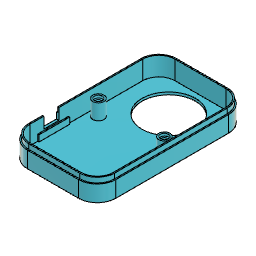
Gehaeuse_unten (Autodesk Fusion 360 design; units mm, degrees)
Autodesk Fusion 360 part; units mm, degrees
note: some values were not read from the file. Set by a fixed rule: which face or edge a step refers to.
sketch "Skizze1" plane through (0, 0, 0) normal (0, 0, 1) x (1, 0, 0)
  circle A0 centre (0, 0) radius 32.5
  circle A1 centre (0, 58.5) radius 21.5
  arc A2 (20.5, -34.5) -> (35.5, -19.5) centre (20.5, -19.5) ccw
  line L0 (35.5, -19.5) -> (35.5, 71)
  arc A3 (35.5, 71) -> (20.5, 86) centre (20.5, 71) ccw
  line L1 (20.5, 86) -> (-20.5, 86)
  arc A4 (-20.5, 86) -> (-35.5, 71) centre (-20.5, 71) ccw
  line L2 (-35.5, 71) -> (-35.5, -19.5)
  arc A5 (-35.5, -19.5) -> (-20.5, -34.5) centre (-20.5, -19.5) ccw
  line L3 (-20.5, -34.5) -> (20.5, -34.5)
extrude "Extrusion1" add sketch "Skizze1" along normal blind 17 contours A0 | A2 L0 A3 L1 A4 L2 A5 L3
shell "Schale1" thickness 2 removed faces 1 at (0.5356, -10.6466, 17)
extrude "Extrusion2" cut 1 faces at (22.6658, 60.7356, 17) along direction (0, 0, -1) up to surface (15 mm away)
sketch "Skizze2" plane through (0, 0, 17) normal (0, 0, 1) x (-1, 0, 0)
  line L0 (20.5, 34.5) -> (-20.5, 34.5)
  arc A0 (-20.5, 34.5) -> (-35.5, 19.5) centre (-20.5, 19.5) ccw
  line L1 (-35.5, 19.5) -> (-35.5, -71)
  arc A1 (-35.5, -71) -> (-20.5, -86) centre (-20.5, -71) ccw
  line L2 (-20.5, -86) -> (20.5, -86)
  arc A2 (20.5, -86) -> (35.5, -71) centre (20.5, -71) ccw
  line L3 (35.5, -71) -> (35.5, 19.5)
  arc A3 (35.5, 19.5) -> (20.5, 34.5) centre (20.5, 19.5) ccw
  arc A4 (33.5, 19.5) -> (20.5, 32.5) centre (20.5, 19.5) ccw
  line L4 (33.5, 19.5) -> (33.5, -71)
  arc A5 (20.5, -84) -> (33.5, -71) centre (20.5, -71) ccw
  line L5 (20.5, -84) -> (-20.5, -84)
  arc A6 (-33.5, -71) -> (-20.5, -84) centre (-20.5, -71) ccw
  line L6 (-33.5, -71) -> (-33.5, 19.5)
  arc A7 (-20.5, 32.5) -> (-33.5, 19.5) centre (-20.5, 19.5) ccw
  line L7 (-20.5, 32.5) -> (20.5, 32.5)
  line L8 (34.5, 19.5) -> (34.5, -71)
  arc A8 (20.5, -85) -> (34.5, -71) centre (20.5, -71) ccw
  line L9 (20.5, -85) -> (-20.5, -85)
  arc A9 (-34.5, -71) -> (-20.5, -85) centre (-20.5, -71) ccw
  line L10 (-34.5, -71) -> (-34.5, 19.5)
  arc A10 (-20.5, 33.5) -> (-34.5, 19.5) centre (-20.5, 19.5) ccw
  line L11 (-20.5, 33.5) -> (20.5, 33.5)
  arc A11 (34.5, 19.5) -> (20.5, 33.5) centre (20.5, 19.5) ccw
  dimension "d32" = 1
extrude "Extrusion3" cut sketch "Skizze2" against normal blind 4 contours L0 A0 L1 A1 L2 A2 L3 A3
sketch "Skizze3" plane through (0, 0, 17) normal (0, 0, 1) x (-1, 0, 0)
  line L0 (-20.5, -85) -> (20.5, -85)
  arc A0 (20.5, -85) -> (34.5, -71) centre (20.5, -71) ccw
  line L1 (34.5, -71) -> (34.5, 19.5)
  arc A1 (34.5, 19.5) -> (20.5, 33.5) centre (20.5, 19.5) ccw
  line L2 (20.5, 33.5) -> (-20.5, 33.5)
  arc A2 (-20.5, 33.5) -> (-34.5, 19.5) centre (-20.5, 19.5) ccw
  line L3 (-34.5, 19.5) -> (-34.5, -71)
  arc A3 (-34.5, -71) -> (-20.5, -85) centre (-20.5, -71) ccw
  arc A4 (33.5, 19.5) -> (20.5, 32.5) centre (20.5, 19.5) ccw
  line L4 (33.5, 19.5) -> (33.5, -71)
  arc A5 (20.5, -84) -> (33.5, -71) centre (20.5, -71) ccw
  line L5 (20.5, -84) -> (-20.5, -84)
  arc A6 (-33.5, -71) -> (-20.5, -84) centre (-20.5, -71) ccw
  line L6 (-33.5, -71) -> (-33.5, 19.5)
  arc A7 (-20.5, 32.5) -> (-33.5, 19.5) centre (-20.5, 19.5) ccw
  line L7 (-20.5, 32.5) -> (20.5, 32.5)
  line L8 (35.5, -3.75) -> (33.5, -3.75)
  line L9 (33.5, 8.25) -> (35.5, 8.25)
  line L10 (33.5, 19.5) -> (33.5, -71)
  line L11 (35.5, 19.5) -> (35.5, -71)
  line L12 (-20.5, 34.5) -> (20.5, 34.5)
  dimension "d36" = 12
  dimension "d37" = 26.25
  constraint horizontal L8
  constraint horizontal L9
  constraint coincident L4 L8.end
  constraint coincident L4 L9.start
  constraint coincident L11 L9.end
  constraint coincident L11 L8.start
  measures "d36" distance of L8 L9
  measures "d37" distance of L9 L12
extrude "Extrusion4" cut sketch "Skizze3" against normal blind 9 contours L1 L4 L8 L9 L10 | L1 L8 L9 L11
sketch "Skizze4" plane through (0, 0, 2) normal (0, 0, 1) x (-1, 0, 0)
  circle A0 centre (0, -58.5) radius 21.5
  line L0 (20.5, 32.5) -> (-20.5, 32.5)
  arc A1 (-20.5, 32.5) -> (-33.5, 19.5) centre (-20.5, 19.5) ccw
  line L1 (-33.5, 19.5) -> (-33.5, -71)
  arc A2 (-33.5, -71) -> (-20.5, -84) centre (-20.5, -71) ccw
  line L2 (-20.5, -84) -> (20.5, -84)
  arc A3 (20.5, -84) -> (33.5, -71) centre (20.5, -71) ccw
  line L3 (33.5, -71) -> (33.5, 19.5)
  arc A4 (33.5, 19.5) -> (20.5, 32.5) centre (20.5, 19.5) ccw
  circle A5 centre (26.5, -28.5) radius 4.5
  circle A6 centre (-26.5, -28.5) radius 4.5
  line L4 (35.5, -3.75) -> (35.5, -71)
  line L5 (-35.5, -71) -> (-35.5, 19.5)
  line L6 (-20.5, 34.5) -> (20.5, 34.5)
  line L7 (20.5, -86) -> (-20.5, -86)
  circle A7 centre (26.5, -28.5) radius 1.75
  circle A8 centre (-26.5, -28.5) radius 1.75
  dimension "d40" = 9
  dimension "d41" = 9
  dimension "d42" = 9
  dimension "d44" = 57.5
  dimension "d45" = 3.5
  constraint equal A5 A6
  constraint horizontal A5.centre A6.centre
  constraint concentric A5 A7
  constraint concentric A6 A8
  constraint equal A7 A8
  measures "d40" diameter of A5
  measures "d41" distance of A5.centre L4
  measures "d42" distance of A6.centre L5
  measures "d44" distance of A5.centre L7
  measures "d45" diameter of A7
extrude "Extrusion5" add sketch "Skizze4" along normal blind 12.5 contours A5 | A6
sketch "Skizze5" plane through (0, 0, 14.5) normal (0, 0, 1) x (-1, 0, 0)
  circle A0 centre (26.5, -28.5) radius 1.75
  circle A1 centre (26.5, -28.5) radius 4.5
sketch "Skizze6" plane through (0, 0, 14.5) normal (0, 0, 1) x (-1, 0, 0)
  circle A0 centre (-26.5, -28.5) radius 1.75
  circle A1 centre (-26.5, -28.5) radius 4.5
  circle A2 centre (26.5, -28.5) radius 1.75
  circle A3 centre (26.5, -28.5) radius 4.5
  circle A4 centre (26.5, -28.5) radius 3.2
  circle A5 centre (-26.5, -28.5) radius 3.2
  dimension "d48" = 6.4
  dimension "d49" = 6.4
  constraint concentric A2 A4
  constraint concentric A0 A5
  measures "d48" diameter of A4
  measures "d49" diameter of A5
extrude "Extrusion6" cut sketch "Skizze6" against normal blind 2 contours A4 | A5
sketch "Skizze8" plane through (0, 0, 2) normal (0, 0, 1) x (-1, 0, 0)
  circle A0 centre (26.5, -28.5) radius 4.5
  circle A1 centre (0, -58.5) radius 21.5
  line L0 (20.5, 32.5) -> (-20.5, 32.5)
  arc A2 (-20.5, 32.5) -> (-33.5, 19.5) centre (-20.5, 19.5) ccw
  line L1 (-33.5, 19.5) -> (-33.5, -71)
  arc A3 (-33.5, -71) -> (-20.5, -84) centre (-20.5, -71) ccw
  line L2 (-20.5, -84) -> (20.5, -84)
  arc A4 (20.5, -84) -> (33.5, -71) centre (20.5, -71) ccw
  line L3 (33.5, -71) -> (33.5, 19.5)
  arc A5 (33.5, 19.5) -> (20.5, 32.5) centre (20.5, 19.5) ccw
  circle A6 centre (-26.5, -28.5) radius 4.5
  line L4 (33.5, -11.5) -> (32.5, -11.5)
  line L5 (32.5, -11.5) -> (32.5, 13.25)
  line L6 (32.5, 13.25) -> (33.5, 13.25)
  line L7 (33.5, 13.25) -> (33.5, -11.5)
  line L8 (35.5, -3.75) -> (35.5, -71)
  line L9 (35.5, -71) -> (35.5, 19.5)
  line L10 (35.5, 19.5) -> (35.5, 8.25)
  line L11 (35.5, 8.25) -> (35.5, -3.75)
  dimension "d230" = 3
  dimension "d231" = 7.75
  dimension "d232" = 5
  constraint horizontal L4
  constraint vertical L5
  constraint horizontal L6
  constraint vertical L7
  constraint coincident L3 L4.start
  measures "d230" distance of L5 L9
  measures "d231" distance of L4 L8.start
  measures "d232" distance of L6 L10.end
extrude "Extrusion8" add sketch "Skizze8" along normal blind 5 contours L3 L4 L5 L6 L7
equation "d41 = 13.5 mm - ( d40 / 2 )"
equation "d42 = d41"
equation "d44 = 62 mm - ( d40 / 2 )"
equation "d49 = d48"
